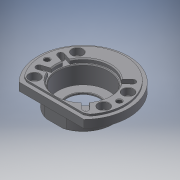
# Autodesk Inventor part: ESR80MP-M
Saved by Autodesk Inventor 2018 (Build 220112000, 112)
## iProperties
Created: 2011-11-01
Part Number: ESR80MP-M
Material: 一般
Document SubType Name: Modeling
Designer: Eric
Density: 1 g/cm^3
Appearance: 預設
Author: Eric
Autodesk Inventor part; units mm, degrees
ref_plane "YZ Plane" through (0, 0, 0) normal (1, 0, 0) x (0, 1, 0)
ref_plane "XZ Plane" through (0, 0, 0) normal (0, 1, 0) x (-1, 0, 0)
ref_plane "XY Plane" through (0, 0, 0) normal (0, 0, 1) x (1, 0, 0)
sketch "草圖1" plane through (0, 0, 0) normal (0, 0, 1) x (1, 0, 0)
  circle A0 centre (0, 0) radius 31
  dimension "d0" = 62
  constraints: 1 centre point, 1 coincident
  measures "d0" diameter of A0
extrude "擠出1" add sketch "草圖1" along normal blind 12.5
sketch "草圖2" plane through (0, 0, 0) normal (0, 0, -1) x (-1, 0, 0)
  circle A0 centre (0, 0) radius 31 projected
  circle A1 centre (0, 0) radius 46.5
  dimension "d3" = 93
  constraints: 1 centre point, 1 coincident
  measures "d3" diameter of A1
extrude "擠出2" add sketch "草圖2" along normal blind 11.85 contours A0 | A1
sketch "草圖3" plane through (0, 0, 0) normal (0, 0, 1) x (1, 0, 0)
  circle A0 centre (0, 0) radius 46.5 projected
  line L0 (0, 46.5) -> (0, -32.6) construction
  line L1 (-33.1586, -32.6) -> (33.1586, -32.6)
  dimension "d6" = 79.1
  constraints: 4 end point, 3 point on circle, 1 perpendicular, 1 vertical
  measures "d6" distance of L0.start L0.end
extrude "擠出3" cut sketch "草圖3" against normal through all contours L1 A0 picked at (8.6933, -34.566)
sketch "草圖4" plane through (0, 0, 12.5) normal (0, 0, 1) x (1, 0, 0)
  circle A0 centre (0, 0) radius 31 projected
  line L0 (0, 31) -> (0, -28.85) construction
  line L1 (-11.3436, -28.85) -> (11.3436, -28.85)
  dimension "d9" = 59.85
  constraints: 4 end point, 3 point on circle, 1 perpendicular, 1 vertical
  measures "d9" distance of L0.start L0.end
extrude "擠出4" cut sketch "草圖4" against normal up to surface (12.5 mm away) contours L1 A0 picked at (-1.287, -29.4862)
sketch "草圖5" plane through (0, 0, 0) normal (0, 0, 1) x (1, 0, 0)
  line L0 (-33.1586, -32.6) -> (33.1586, -32.6) projected
  arc A0 (33.1586, -32.6) -> (-33.1586, -32.6) centre (0, 0) ccw projected
  arc A1 (11.3436, -28.85) -> (-11.3436, -28.85) centre (0, 0) ccw projected
  line L1 (-11.3436, -28.85) -> (11.3436, -28.85) projected
  arc A2 (33.5596, -26.7238) -> (-33.5596, -26.7238) centre (0, 0) ccw
  line L2 (-29, -28.85) -> (29, -28.85)
  line L3 (-29, -28.85) -> (-33.5596, -26.7238)
  line L4 (0, 0) -> (0, -43.8205) construction
  line L5 (29, -28.85) -> (33.5596, -26.7238)
  dimension "d12" = 85.8
  dimension "d91" = 29
  dimension "d144" = 25
  constraints: 8 end point, 2 point on circle, 2 symmetric about line, 1 centre point, 1 coincident, 1 collinear, 1 horizontal, 1 perpendicular
  measures "d12" diameter of A2
  measures "d91" horizontal distance of L2.start A0.centre
  measures "d144" angle of L2 L3
extrude "擠出5" cut sketch "草圖5" against normal blind 1.9
sketch "草圖6" plane through (0, 0, -11.85) normal (0, 0, -1) x (-1, 0, 0)
  line L0 (-33.1586, -32.6) -> (33.1586, -32.6) projected
  arc A0 (33.1586, -32.6) -> (-33.1586, -32.6) centre (0, 0) ccw projected
  arc A1 (33.5596, -26.7238) -> (-33.5596, -26.7238) centre (0, 0) ccw projected
  line L1 (29, -28.85) -> (-29, -28.85) projected
  line L2 (-29, -28.85) -> (-33.5596, -26.7238) projected
  line L3 (33.5596, -26.7238) -> (29, -28.85) projected
extrude "擠出6" cut sketch "草圖6" against normal blind 1.9
sketch "草圖8" plane through (0, 0, -11.85) normal (0, 0, -1) x (-1, 0, 0)
  arc A0 (33.5596, -26.7238) -> (-33.5596, -26.7238) centre (0, 0) ccw projected
  circle A1 centre (0, 0) radius 26
  point P0 (-31.5474, -28.85)
  point P1 (31.5474, -28.85)
  dimension "d56" = 52
  constraints: 1 centre point, 1 coincident, 1 other
  measures "d56" diameter of A1
extrude "擠出7" cut sketch "草圖8" against normal blind 22.5
sketch "草圖9" plane through (0, 0, -11.85) normal (0, 0, -1) x (-1, 0, 0)
  circle A0 centre (0, 0) radius 26 projected
  arc A1 (33.5596, -26.7238) -> (-33.5596, -26.7238) centre (0, 0) ccw projected
  circle A2 centre (0, 0) radius 27.5
  point P0 (-31.5474, -28.85)
  point P1 (31.5474, -28.85)
  dimension "d57" = 55
  constraints: 1 centre point, 1 coincident, 1 other
  measures "d57" diameter of A2
extrude "擠出8" [suppressed]
sketch "草圖11" plane through (0, 0, 12.5) normal (0, 0, 1) x (1, 0, 0)
  arc A0 (11.3436, -28.85) -> (-11.3436, -28.85) centre (0, 0) ccw projected
  circle A1 centre (0, 0) radius 16.5
  dimension "d60" = 33
  constraints: 1 centre point, 1 coincident
  measures "d60" diameter of A1
extrude "擠出9" cut sketch "草圖11" against normal through all
sketch "草圖7" plane through (0, 0, -11.85) normal (0, 0, -1) x (-1, 0, 0)
  line L0 (-29, -28.85) -> (29, -28.85) projected
  arc A0 (33.5596, -26.7238) -> (-33.5596, -26.7238) centre (0, 0) ccw projected
  line L1 (-11.8355, 0) -> (18.8816, 0) construction
  line L2 (0, 11.001) -> (0, -17.2637) construction
  point P0 (-37, 0)
  point P1 (37, 0)
  point P2 (-33.5, 12.5)
  point P3 (-33.5, -12.5)
  point P4 (28, 22)
  point P5 (28, -22)
  point P6 (34.24, -11.12)
  point P7 (34.24, 11.12)
  point P8 (-26.75, 24.1)
  point P9 (-26.75, -24.1)
  point P10 (-33.5, -12.5)
  point P11 (-33.5, 12.5)
  dimension "d17" = 37
  dimension "d18" = 37
  dimension "d93" = 12.5
  dimension "d95" = 33.5
  dimension "d96" = 33.5
  dimension "d97" = 22
  dimension "d98" = 28
  dimension "d99" = 28
  dimension "d100" = 22
  dimension "d101" = 11.12
  dimension "d102" = 11.12
  dimension "d103" = 12.5
  dimension "d104" = 24.1
  dimension "d105" = 24.1
  dimension "d106" = 26.75
  dimension "d107" = 26.75
  dimension "d108" = 34.24
  dimension "d109" = 34.24
  constraints: 4 end point, 2 coincident, 1 parallel, 1 perpendicular, 1 vertical
  measures "d17" distance of A0.centre point (-37, 0)
  measures "d18" distance of A0.centre point (37, 0)
  measures "d93" vertical distance of A0.centre point (-33.5, 12.5)
  measures "d95" horizontal distance of A0.centre point (-33.5, 12.5)
  measures "d96" horizontal distance of A0.centre point (-33.5, -12.5)
  measures "d97" vertical distance of point (28, 22) A0.centre
  measures "d98" horizontal distance of point (28, 22) A0.centre
  measures "d99" horizontal distance of point (28, -22) A0.centre
  measures "d100" vertical distance of point (28, -22) A0.centre
  measures "d101" vertical distance of A0.centre point (34.24, 11.12)
  measures "d102" vertical distance of point (34.24, -11.12) A0.centre
  measures "d103" vertical distance of A0.centre point (-33.5, -12.5)
  measures "d104" vertical distance of A0.centre point (-26.75, 24.1)
  measures "d105" vertical distance of A0.centre point (-26.75, -24.1)
  measures "d106" horizontal distance of A0.centre point (-26.75, -24.1)
  measures "d107" horizontal distance of A0.centre point (-26.75, 24.1)
  measures "d108" horizontal distance of A0.centre point (34.24, -11.12)
  measures "d109" horizontal distance of A0.centre point (34.24, 11.12)
hole "孔1" at (37, 0, -11.85) at (-37, 0, -11.85) direction (0, 0, 1) diameter 4.917 end through all thread size "M6x1" class "6H" standard "ISO Metric profile"
hole "孔2" at (-28, 22, -11.85) at (-28, -22, -11.85) at (33.5, -12.5, -11.85) at (33.5, 12.5, -11.85) direction (0, 0, 1) diameter 6.8 end through all counterbore diameter 11 counterbore depth 7
hole "孔3" at (-34.24, -11.12, -11.85) at (-34.24, 11.12, -11.85) at (26.75, 24.1, -11.85) at (26.75, -24.1, -11.85) direction (0, 0, 1) diameter 6 end through all
chamfer "倒角1" distance 0.5 angle 45 4 edges at (37, -2.4585, -11.85) (-37, -2.4585, -11.85) (-37, -2.4585, 0) (37, -2.4585, 0)
chamfer "倒角2" distance 0.3 angle 45 16 edges at (-28, -25.4, 0) (-34.24, -14.12, 0) (-34.24, 8.12, 0) (-28, 18.6, 0) (26.75, 21.1, 0) (33.5, 9.1, 0) (33.5, -15.9, 0) (26.75, -27.1, 0) (33.5, 7, -11.85) (33.5, -18, -11.85) (-28, -27.5, -11.85) (-28, 16.5, -11.85) (-28, 18.6, -4.85) (33.5, 9.1, -4.85) (33.5, -15.9, -4.85) (-28, -25.4, -4.85)
chamfer "倒角3" [suppressed]
chamfer "倒角4" [suppressed]
chamfer "倒角5" distance 0.5 angle 45 1 edges at (-16.5, 0, 10.65)
sketch "草圖14" plane through (0, 0, -11.85) normal (0, 0, -1) x (-1, 0, 0)
  circle A0 centre (34.24, -11.12) radius 3 projected
  circle A1 centre (34.24, 11.12) radius 3 projected
  circle A2 centre (-26.75, 24.1) radius 3 projected
  circle A3 centre (-26.75, -24.1) radius 3 projected
  line L0 (-26.75, -24.1) -> (0, 0) construction
  line L1 (34.24, -11.12) -> (0, 0) construction
  line L2 (34.24, 11.12) -> (0, 0) construction
  line L3 (-26.75, 24.1) -> (0, 0) construction
  line L4 (-24.742, 26.3288) -> (-17.1796, 19.5157)
  line L5 (-28.758, 21.8712) -> (-21.1957, 15.058)
  line L6 (33.3133, 13.9733) -> (23.6368, 10.8307)
  line L7 (35.1667, 8.2667) -> (25.4901, 5.1241)
  line L8 (35.1667, -8.2667) -> (25.4901, -5.1241)
  line L9 (33.3133, -13.9733) -> (23.6368, -10.8307)
  line L10 (-24.742, -26.3288) -> (-17.1796, -19.5157)
  line L11 (-28.758, -21.8712) -> (-21.1957, -15.058)
  arc A4 (-24.742, 26.3288) -> (-28.758, 21.8712) centre (-26.75, 24.1) ccw
  arc A5 (35.1667, 8.2667) -> (33.3133, 13.9733) centre (34.24, 11.12) ccw
  arc A6 (33.3133, -13.9733) -> (35.1667, -8.2667) centre (34.24, -11.12) ccw
  arc A7 (-28.758, -21.8712) -> (-24.742, -26.3288) centre (-26.75, -24.1) ccw
  arc A8 (-17.1796, 19.5157) -> (-21.1957, 15.058) centre (0, 0) ccw
  circle A9 centre (0, 0) radius 26 projected
  dimension "d111" = 3
  dimension "d117" = 3
  dimension "d118" = 3
  dimension "d119" = 3
  dimension "d120" = 3
  dimension "d121" = 3
  dimension "d122" = 3
  dimension "d123" = 3
  dimension "d124" = 6
  dimension "d125" = 6
  dimension "d126" = 6
  constraints: 24 end point, 16 point on circle, 8 parallel, 5 centre point, 4 coincident
  measures "d111" distance between parallel lines of L4 L3
  measures "d117" distance between parallel lines of L6 L2
  measures "d118" distance between parallel lines of L5 L3
  measures "d119" distance between parallel lines of L10 L0
  measures "d120" distance between parallel lines of L11 L0
  measures "d121" distance between parallel lines of L9 L1
  measures "d122" distance between parallel lines of L1 L8
  measures "d123" distance between parallel lines of L7 L2
  measures "d124" diameter of A5
  measures "d125" diameter of A6
  measures "d126" diameter of A7
extrude "擠出11" [suppressed]
feature "Alias Freeform1" [suppressed]
mirror "鏡射1" about plane through (0, 0, -11.85) normal (0, 0, -1) remove original yes
extrude "擠出13" cut sketch "草圖14" along normal blind 4 contours L5 A2 L4 A8
extrude "擠出14" cut sketch "草圖14" along normal blind 4 contours A0 L9 A9 L8 | L10 A3 L11 A9 | A9 L6 A1 L7
sketch "草圖15" plane through (0, 0, -11.85) normal (0, 0, 1) x (1, 0, 0)
  arc A0 (33.5596, -26.7238) -> (-33.5596, -26.7238) centre (0, 0) ccw projected
  circle A1 centre (0, 0) radius 27.5
  dimension "d138" = 55
  constraints: 1 centre point, 1 coincident
  measures "d138" diameter of A1
extrude "擠出15" cut sketch "草圖15" against normal blind 4
chamfer "倒角6" distance 1 angle 45 4 edges at (-5.7234, 26.8978, -11.85) (-27.5, 0, -11.85) (-5.7234, -26.8978, -11.85) (27.5, 0, -11.85)
chamfer "倒角7" distance 1 angle 30 1 edges at (26, 0, -15.85) measured on face at (26, 0, -16.35)
chamfer "倒角8" distance 1 angle 45 1 edges at (0, 31, -36.2)
